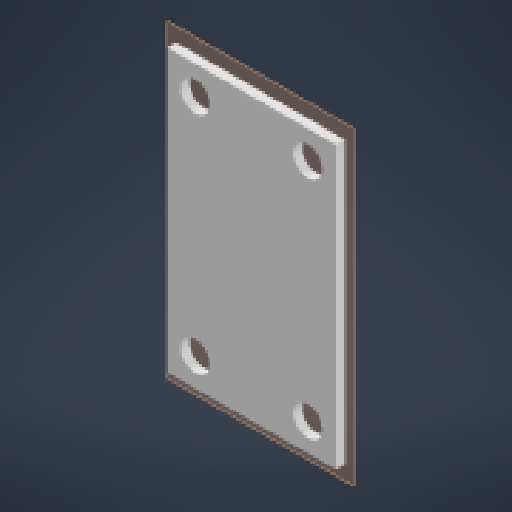
# Autodesk Inventor part: top
Saved by Autodesk Inventor 2027 (Build 310192060, 192F)
## iProperties
Created: 2026-05-29
Part Number: top
Material: Generic
Document SubType Name: Modeling
Designer: jacob
Density: 1 g/cm^3
Appearance: Default
Author: jacob
Autodesk Inventor part; units mm, degrees
ref_plane "YZ Plane" through (0, 0, 0) normal (1, 0, 0) x (0, 1, 0)
ref_plane "XZ Plane" through (0, 0, 0) normal (0, 1, 0) x (-1, 0, 0)
ref_plane "XY Plane" through (0, 0, 0) normal (0, 0, 1) x (1, 0, 0)
ref_plane "Work Plane2" through (-0.0135, 12.5, 0) normal (0, 0, 1) x (1, 0, 0)
sketch "Sketch7" plane through (-0.0135, 12.5, 0) normal (0, 0, 1) x (1, 0, 0)
  circle A0 centre (12.4731, -25.0135) radius 3.25 projected
  circle A1 centre (-12.5269, -25.0135) radius 3.25 projected
  circle A2 centre (12.4731, 24.9865) radius 3.25 projected
  circle A3 centre (-12.5269, 24.9865) radius 3.25 projected
  line L0 (18.7837, -31.2297) -> (18.7163, 31.2702) projected
  line L1 (18.7163, 31.2702) -> (-18.7837, 31.2297) projected
  line L2 (-18.7837, 31.2297) -> (-18.7163, -31.2702) projected
  line L3 (-18.7163, -31.2702) -> (18.7837, -31.2297) projected
  point P0 (0.0135, -12.5)
extrude "Extrusion3" add sketch "Sketch7" along normal blind 2
body "Solid2"
